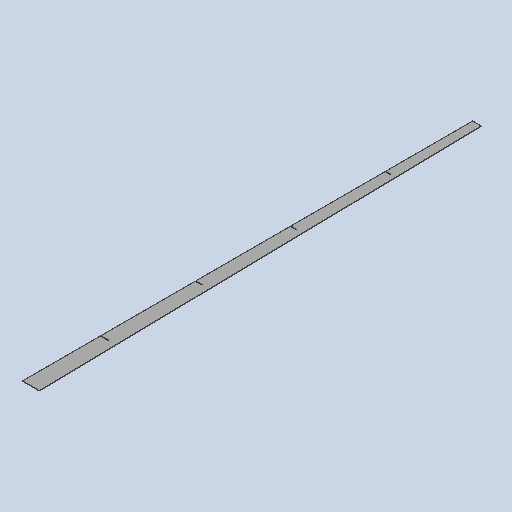
# Autodesk Inventor part: BSH 022 rib board
Saved by Autodesk Inventor 2025 (Build 290162010, 162A)
## iProperties
Created: 2024-07-23
Part Number: BSH 022 rib board
Material: 09g2s
Document SubType Name: Sheet Metal
Designer: admin
Density: 7.85 g/cm^3
Sheet Metal Rule: AISI304 3mm Die 32
Appearance: Default
Mass: 4739.97 g
Surface Area: 4201.54 cm^2
Volume: 603.817 cm^3
Flat Pattern Width: 9.91654 cm
Flat Pattern Length: 265.636 cm
Flat Pattern Area: 2634.2 cm^2
Sheet Metal Width: 99,165 mm
Sheet Metal Length: 2656,364 mm
Sheet Metal Area: 263419,502 mm^2
Stock Number: БШК 022 шпангоут борт
Author: admin
Autodesk Inventor part; units mm, degrees
ref_plane "YZ Plane" through (0, 0, 0) normal (1, 0, 0) x (0, 1, 0)
ref_plane "XZ Plane" through (0, 0, 0) normal (0, 1, 0) x (-1, 0, 0)
ref_plane "XY Plane" through (0, 0, 0) normal (0, 0, 1) x (1, 0, 0)
sketch "Sketch1" plane through (0, 0, 0) normal (0, 0, 1) x (1, 0, 0)
  line L0 (1200, 2950) -> (-1200, 2950)
  line L1 (-1200, 2950) -> (-1200, 0)
  line L2 (-1200, 0) -> (1200, 0)
  line L3 (1200, 0) -> (1200, 2950)
  line L4 (1150, 2950) -> (1150, 0)
  line L5 (-1150, 0) -> (-1150, 2950) construction
  line L6 (0, 2950) -> (0, 50) construction
  line L7 (-1100, 200) -> (-950, 50)
  line L8 (-1200, 100) -> (-1100, 100)
  line L9 (-1100, 100) -> (-1100, 0)
  line L10 (-1100, 200) -> (-1150, 2950)
  arc A0 (-1100.4545, 224.9959) -> (-1082.3223, 182.3223) centre (-1100, 200) ccw
  arc A1 (-1082.3223, 182.3223) -> (-1100.4545, 224.9959) centre (-1100, 200) ccw construction
  line L11 (-1200, 255) -> (-1101, 255) construction
  line L12 (0, 50) -> (-950, 50)
  line L13 (0, 50) -> (0, 0)
  line L14 (1505.3449, -225.894) -> (355.3449, -225.894)
  line L15 (-1200, 245) -> (-1100.8182, 245)
  line L16 (-1200, 2900) -> (-1149.0909, 2900)
  dimension "d3" = 2400
  dimension "d4" = 2950
  dimension "d5" = 50
  dimension "d6" = 100
  dimension "d7" = 50
  dimension "d9" = 135
  dimension "d10" = 950
  dimension "d11" = 1150
  dimension "d12" = 136.042
  dimension "d13" = 50
  dimension "d14" = 100
  dimension "d15" = 212.132
  dimension "d17" = 55
  dimension "d20" = 200
  dimension "d50" = 2705
  dimension "d53" = 50
  measures "d3" distance of L3.start L1.end
  measures "d4" distance of L1.end L1.start
  measures "d5" diameter of A0
  measures "d6" distance of L8.start L8.end
  measures "d7" distance between parallel lines of L1 L5
  measures "d9" angle of L12 L7
  measures "d10" distance of L6.end L7.end
  measures "d11" distance of L14.start L14.end
  measures "d12" angle of L7 L10
  measures "d13" distance between parallel lines of L2 L12
  measures "d14" distance from line of L1 L10.start
  measures "d15" distance of L10.start L7.end
  measures "d17" vertical distance of L10.start L11.end
  measures "d20" distance from line of L2 A1.centre
  measures "d50" distance of L1.start L15.start
  measures "d53" distance of L16.start L1.start
extrude "Plate1" add sketch "Sketch1" along normal blind 3 contours L10 L15 L1 L16
sketch "Sketch2" plane through (0, 0, 3) normal (0, 0, 1) x (1, 0, 0)
  line L0 (-1149.0909, 2900) -> (-1100.8182, 245) projected
  line L1 (-1200, 245) -> (-1200, 2900) projected
  line L2 (-1100.8182, 245) -> (-1150, 2950) projected
  line L3 (-1158.8362, 1267.3142) -> (-1158.778, 1264.1148)
  line L4 (-1158.778, 1264.1148) -> (-1119.3606, 1264.8314) construction
  line L5 (-1150, 2950) -> (-1100.8182, 245) projected
  line L6 (-1158.778, 1264.1148) -> (-1200, 1263.3653)
  line L7 (-1158.8362, 1267.3142) -> (-1200, 1266.5658)
  line L8 (-1200, 703.2727) -> (-1153.6813, 704.1149)
  line L9 (-1153.6813, 704.1149) -> (-1153.7395, 707.3144)
  line L10 (-1153.6813, 704.1149) -> (-1109.1804, 704.924) construction
  line L11 (-1153.7395, 707.3144) -> (-1200, 706.4732)
  line L12 (-1200, 1823.4578) -> (-1163.8614, 1824.1149)
  line L13 (-1163.8614, 1824.1149) -> (-1163.9196, 1827.3144)
  line L14 (-1163.9196, 1827.3144) -> (-1200, 1826.6584)
  line L15 (-1163.8614, 1824.1149) -> (-1129.5407, 1824.7389) construction
  line L16 (-1200, 2383.5504) -> (-1168.9515, 2384.1149)
  line L17 (-1168.9515, 2384.1149) -> (-1169.0097, 2387.3144)
  line L18 (-1168.9515, 2384.1149) -> (-1139.7208, 2384.6464) construction
  line L19 (-1169.0097, 2387.3144) -> (-1200, 2386.7509)
  line L20 (-1100.8182, 245) -> (-1200, 245) projected
  line L21 (-1200, 2900) -> (-1149.0909, 2900) projected
  point P0 (0, 0)
  dimension "d34" = 46.3264
  dimension "d36" = 41.2288
  dimension "d39" = 36.1445
  dimension "d42" = 31.0536
  dimension "d43" = 560
  dimension "d44" = 3.2
  dimension "d45" = 560
  dimension "d46" = 3.2
  dimension "d47" = 560
  dimension "d48" = 3.2
  dimension "d49" = 3.2
  dimension "d52" = 460
  constraints: 32 end point, 11 perpendicular, 6 parallel, 4 point on line, 1 collinear, 9 other
  measures "d34" distance of L8.start L8.end
  measures "d36" distance of L6.end L3.end
  measures "d39" distance of L12.start L12.end
  measures "d42" distance of L16.end L16.start
  measures "d43" distance of L4.end L10.end
  measures "d44" distance between parallel lines of L8 L11
  measures "d45" distance of L15.end L4.end
  measures "d46" distance between parallel lines of L6 L7
  measures "d47" distance of L18.end L15.end
  measures "d48" distance between parallel lines of L12 L14
  measures "d49" distance between parallel lines of L16 L19
  measures "d52" distance from line of L0.end L10
extrude "Extrusion1" cut sketch "Sketch2" against normal through all contours L19 L17 L16 L1 | L1 L11 L9 L8 | L14 L13 L12 L1 | L1 L7 L3 L6
equation "\"d11\" = d10 + d18"
equation "\"d14\" = d6"
equation "\"d43\" = Stringer1_step"
equation "\"d45\" = Stringer1_step"
equation "\"d47\" = Stringer1_step"
equation "\"d52\" = Stringer1_hight"
equation "\"d2\" = Thickness"
equation "\"BendReliefWidth\" = Thickness"
equation "\"BendReliefDepth\" = 0.5 * Thickness"
equation "\"CornerReliefSize\" = 4 * Thickness"
equation "\"MinimumRemnant\" = 2 * Thickness"
equation "\"TransitionRadius\" = BendRadius"
equation "\"JacobiRadiusSize\" = BendRadius"
equation "\"GapSize\" = Thickness"
equation "\"d18\" = d19"
equation "\"Stringer1_step\" = 560"
equation "\"Stringer1_hight\" = 460"
equation "\"Thickness\" = 3"
equation "\"BendRadius\" = 5"
equation "\"d19\" = 200"
body "Solid1"
